Autodesk Fusion 360 part; units mm, degrees
(part 3 of 4)
sketch "SupportPlate" plane through (0, 0, 0) normal (0, 0, 1) x (1, 0, 0)
  line L0 (113.5494, -107.4434) -> (117.1134, -109.2589)
  spline S0 degree 3 poles (117.1134, -109.2589) (117.3594, -109.3843) (117.6605, -109.2865) (117.7859, -109.0398) knots 0 0 0 0 1 1 1 1
  line L1 (117.7859, -109.0398) -> (118.013, -108.5947)
  line L2 (118.013, -108.5947) -> (121.5769, -110.4103)
  spline S1 degree 3 poles (121.5769, -110.4103) (121.8229, -110.5362) (122.124, -110.4384) (122.2494, -110.1926) knots 0 0 0 0 1 1 1 1
  line L3 (122.2494, -110.1926) -> (128.1513, -98.6093)
  spline S2 degree 3 poles (128.1513, -98.6093) (128.2766, -98.3632) (128.1788, -98.0621) (127.9328, -97.937) knots 0 0 0 0 1 1 1 1
  line L4 (127.9328, -97.937) -> (124.3688, -96.1196)
  line L5 (124.3688, -96.1196) -> (124.5958, -95.6752)
  spline S3 degree 3 poles (124.5958, -95.6752) (124.7211, -95.4293) (124.6233, -95.1282) (124.3773, -95.0029) knots 0 0 0 0 1 1 1 1
  line L6 (124.3773, -95.0029) -> (120.8133, -93.1874)
  spline S4 degree 3 poles (120.8133, -93.1874) (120.5672, -93.0615) (120.2661, -93.1593) (120.1407, -93.4052) knots 0 0 0 0 1 1 1 1
  line L7 (120.1407, -93.4052) -> (119.9137, -93.8521)
  line L8 (119.9137, -93.8521) -> (116.3497, -92.0347)
  spline S5 degree 3 poles (116.3497, -92.0347) (116.1036, -91.9095) (115.8026, -92.0074) (115.6772, -92.2537) knots 0 0 0 0 1 1 1 1
  line L9 (115.6772, -92.2537) -> (109.7754, -103.837)
  spline S6 degree 3 poles (109.7754, -103.837) (109.6499, -104.0825) (109.7478, -104.3836) (109.9938, -104.5093) knots 0 0 0 0 1 1 1 1
  line L10 (109.9938, -104.5093) -> (113.5579, -106.3246)
  line L11 (113.5579, -106.3246) -> (113.3309, -106.7711)
  spline S7 degree 3 poles (113.3309, -106.7711) (113.2055, -107.0165) (113.3033, -107.3176) (113.5494, -107.4434) knots 0 0 0 0 1 1 1 1
  line L12 (129.9703, -110.4119) -> (133.5342, -112.2274)
  line L13 (133.5342, -112.2274) -> (133.3072, -112.6724)
  spline S8 degree 3 poles (133.3072, -112.6724) (133.1819, -112.9189) (133.2797, -113.22) (133.5258, -113.346) knots 0 0 0 0 1 1 1 1
  line L14 (133.5258, -113.346) -> (137.0897, -115.1615)
  spline S9 degree 3 poles (137.0897, -115.1615) (137.3358, -115.2867) (137.6369, -115.1889) (137.7623, -114.9424) knots 0 0 0 0 1 1 1 1
  line L15 (137.7623, -114.9424) -> (137.9893, -114.4975)
  line L16 (137.9893, -114.4975) -> (141.5533, -116.3129)
  spline S10 degree 3 poles (141.5533, -116.3129) (141.7994, -116.4387) (142.1004, -116.3408) (142.2258, -116.0952) knots 0 0 0 0 1 1 1 1
  line L17 (142.2258, -116.0952) -> (148.1276, -104.5119)
  spline S11 degree 3 poles (148.1276, -104.5119) (148.253, -104.2656) (148.1552, -103.9646) (147.9091, -103.8397) knots 0 0 0 0 1 1 1 1
  line L18 (147.9091, -103.8397) -> (144.3451, -102.0224)
  line L19 (144.3451, -102.0224) -> (144.5721, -101.5778)
  spline S12 degree 3 poles (144.5721, -101.5778) (144.6975, -101.3317) (144.5997, -101.0306) (144.3536, -100.9056) knots 0 0 0 0 1 1 1 1
  line L20 (144.3536, -100.9056) -> (140.7896, -99.0887)
  spline S13 degree 3 poles (140.7896, -99.0887) (140.5436, -98.9639) (140.2425, -99.0617) (140.1171, -99.3078) knots 0 0 0 0 1 1 1 1
  line L21 (140.1171, -99.3078) -> (139.8901, -99.7523)
  line L22 (139.8901, -99.7523) -> (136.3261, -97.9373)
  spline S14 degree 3 poles (136.3261, -97.9373) (136.08, -97.812) (135.779, -97.9098) (135.6536, -98.1564) knots 0 0 0 0 1 1 1 1
  line L23 (135.6536, -98.1564) -> (129.7517, -109.7383)
  spline S15 degree 3 poles (129.7517, -109.7383) (129.6264, -109.985) (129.7242, -110.2861) (129.9703, -110.4119) knots 0 0 0 0 1 1 1 1
  line L24 (99.4151, -97.8124) -> (99.4152, -97.3129)
  line L25 (99.4152, -97.3129) -> (103.4151, -97.3123)
  spline S16 degree 3 poles (103.4151, -97.3123) (103.6912, -97.3118) (103.9151, -97.088) (103.9151, -96.8123) knots 0 0 0 0 1 1 1 1
  line L26 (103.9151, -96.8123) -> (103.9151, -83.8115)
  spline S17 degree 3 poles (103.9151, -83.8115) (103.9151, -83.5357) (103.6912, -83.3118) (103.4151, -83.3114) knots 0 0 0 0 1 1 1 1
  line L27 (103.4151, -83.3114) -> (99.4152, -83.3112)
  line L28 (99.4152, -83.3112) -> (99.4151, -82.8115)
  spline S18 degree 3 poles (99.4151, -82.8115) (99.4151, -82.5358) (99.1912, -82.312) (98.9151, -82.3115) knots 0 0 0 0 1 1 1 1
  line L29 (98.9151, -82.3115) -> (94.9151, -82.3115)
  spline S19 degree 3 poles (94.9151, -82.3115) (94.639, -82.312) (94.4151, -82.5358) (94.4151, -82.8115) knots 0 0 0 0 1 1 1 1
  line L30 (94.4151, -82.8115) -> (94.4151, -83.3112)
  line L31 (94.4151, -83.3112) -> (90.4151, -83.3114)
  spline S20 degree 3 poles (90.4151, -83.3114) (90.139, -83.3117) (89.9151, -83.5357) (89.9151, -83.8115) knots 0 0 0 0 1 1 1 1
  line L32 (89.9151, -83.8115) -> (89.9151, -96.8123)
  spline S21 degree 3 poles (89.9151, -96.8123) (89.9151, -97.088) (90.139, -97.3119) (90.4151, -97.3123) knots 0 0 0 0 1 1 1 1
  line L33 (90.4151, -97.3123) -> (94.4151, -97.3129)
  line L34 (94.4151, -97.3129) -> (94.4151, -97.8124)
  spline S22 degree 3 poles (94.4151, -97.8124) (94.4151, -98.088) (94.639, -98.3119) (94.9151, -98.3124) knots 0 0 0 0 1 1 1 1
  line L35 (94.9151, -98.3124) -> (98.9151, -98.3124)
  spline S23 degree 3 poles (98.9151, -98.3124) (99.1912, -98.3119) (99.4151, -98.088) (99.4151, -97.8124) knots 0 0 0 0 1 1 1 1
  line L36 (61.3151, -97.8124) -> (61.3152, -97.3129)
  line L37 (61.3152, -97.3129) -> (65.3151, -97.3123)
  spline S24 degree 3 poles (65.3151, -97.3123) (65.5912, -97.3118) (65.8151, -97.088) (65.8152, -96.8123) knots 0 0 0 0 1 1 1 1
  line L38 (65.8152, -96.8123) -> (65.8152, -83.8115)
  spline S25 degree 3 poles (65.8152, -83.8115) (65.8151, -83.5357) (65.5912, -83.3118) (65.3151, -83.3114) knots 0 0 0 0 1 1 1 1
  line L39 (65.3151, -83.3114) -> (61.3152, -83.3112)
  line L40 (61.3152, -83.3112) -> (61.3151, -82.8115)
  spline S26 degree 3 poles (61.3151, -82.8115) (61.3151, -82.5358) (61.0912, -82.312) (60.8151, -82.3115) knots 0 0 0 0 1 1 1 1
  line L41 (60.8151, -82.3115) -> (56.8151, -82.3115)
  spline S27 degree 3 poles (56.8151, -82.3115) (56.539, -82.312) (56.3151, -82.5358) (56.3151, -82.8115) knots 0 0 0 0 1 1 1 1
  line L42 (56.3151, -82.8115) -> (56.3151, -83.3112)
  line L43 (56.3151, -83.3112) -> (52.3151, -83.3114)
  spline S28 degree 3 poles (52.3151, -83.3114) (52.039, -83.3117) (51.8151, -83.5357) (51.8151, -83.8115) knots 0 0 0 0 1 1 1 1
  line L44 (51.8151, -83.8115) -> (51.8151, -96.8123)
  spline S29 degree 3 poles (51.8151, -96.8123) (51.8151, -97.088) (52.039, -97.3119) (52.3151, -97.3123) knots 0 0 0 0 1 1 1 1
  line L45 (52.3151, -97.3123) -> (56.3151, -97.3129)
  line L46 (56.3151, -97.3129) -> (56.3151, -97.8124)
  spline S30 degree 3 poles (56.3151, -97.8124) (56.3151, -98.088) (56.539, -98.3119) (56.8151, -98.3124) knots 0 0 0 0 1 1 1 1
  line L47 (56.8151, -98.3124) -> (60.8151, -98.3124)
  spline S31 degree 3 poles (60.8151, -98.3124) (61.0912, -98.3119) (61.3151, -98.088) (61.3151, -97.8124) knots 0 0 0 0 1 1 1 1
  line L48 (80.3651, -95.4312) -> (80.3652, -94.9316)
  line L49 (80.3652, -94.9316) -> (84.3651, -94.9311)
  spline S32 degree 3 poles (84.3651, -94.9311) (84.6412, -94.9305) (84.8651, -94.7067) (84.8652, -94.431) knots 0 0 0 0 1 1 1 1
  line L50 (84.8652, -94.431) -> (84.8652, -81.4302)
  spline S33 degree 3 poles (84.8652, -81.4302) (84.8651, -81.1545) (84.6413, -80.9306) (84.3651, -80.9302) knots 0 0 0 0 1 1 1 1
  line L51 (84.3651, -80.9302) -> (80.3652, -80.9299)
  line L52 (80.3652, -80.9299) -> (80.3651, -80.4303)
  spline S34 degree 3 poles (80.3651, -80.4303) (80.3651, -80.1546) (80.1412, -79.9307) (79.8651, -79.9303) knots 0 0 0 0 1 1 1 1
  line L53 (79.8651, -79.9303) -> (75.8651, -79.9303)
  spline S35 degree 3 poles (75.8651, -79.9303) (75.589, -79.9308) (75.3651, -80.1546) (75.3651, -80.4303) knots 0 0 0 0 1 1 1 1
  line L54 (75.3651, -80.4303) -> (75.3651, -80.9299)
  line L55 (75.3651, -80.9299) -> (71.3651, -80.9302)
  spline S36 degree 3 poles (71.3651, -80.9302) (71.089, -80.9305) (70.8651, -81.1545) (70.8651, -81.4302) knots 0 0 0 0 1 1 1 1
  line L56 (70.8651, -81.4302) -> (70.8651, -94.431)
  spline S37 degree 3 poles (70.8651, -94.431) (70.8651, -94.7067) (71.089, -94.9306) (71.3651, -94.9311) knots 0 0 0 0 1 1 1 1
  line L57 (71.3651, -94.9311) -> (75.3651, -94.9316)
  line L58 (75.3651, -94.9316) -> (75.3651, -95.4312)
  spline S38 degree 3 poles (75.3651, -95.4312) (75.3651, -95.7068) (75.589, -95.9306) (75.8651, -95.9312) knots 0 0 0 0 1 1 1 1
  line L59 (75.8651, -95.9312) -> (79.8651, -95.9312)
  spline S39 degree 3 poles (79.8651, -95.9312) (80.1412, -95.9307) (80.3651, -95.7068) (80.3651, -95.4312) knots 0 0 0 0 1 1 1 1
  line L60 (42.2651, -83.5249) -> (42.2652, -83.0254)
  line L61 (42.2652, -83.0254) -> (46.2651, -83.0248)
  spline S40 degree 3 poles (46.2651, -83.0248) (46.5412, -83.0243) (46.7651, -82.8005) (46.7651, -82.5248) knots 0 0 0 0 1 1 1 1
  line L62 (46.7651, -82.5248) -> (46.7651, -69.524)
  spline S41 degree 3 poles (46.7651, -69.524) (46.7651, -69.2482) (46.5412, -69.0243) (46.2651, -69.0239) knots 0 0 0 0 1 1 1 1
  line L63 (46.2651, -69.0239) -> (42.2652, -69.0237)
  line L64 (42.2652, -69.0237) -> (42.2651, -68.524)
  spline S42 degree 3 poles (42.2651, -68.524) (42.2651, -68.2483) (42.0412, -68.0245) (41.7651, -68.024) knots 0 0 0 0 1 1 1 1
  line L65 (41.7651, -68.024) -> (37.7651, -68.024)
  spline S43 degree 3 poles (37.7651, -68.024) (37.489, -68.0245) (37.2651, -68.2483) (37.2651, -68.524) knots 0 0 0 0 1 1 1 1
  line L66 (37.2651, -68.524) -> (37.2651, -69.0237)
  line L67 (37.2651, -69.0237) -> (33.2651, -69.0239)
  spline S44 degree 3 poles (33.2651, -69.0239) (32.989, -69.0242) (32.7651, -69.2482) (32.7651, -69.524) knots 0 0 0 0 1 1 1 1
  line L68 (32.7651, -69.524) -> (32.7651, -82.5248)
  spline S45 degree 3 poles (32.7651, -82.5248) (32.7651, -82.8005) (32.989, -83.0244) (33.2651, -83.0248) knots 0 0 0 0 1 1 1 1
  line L69 (33.2651, -83.0248) -> (37.2651, -83.0254)
  line L70 (37.2651, -83.0254) -> (37.2651, -83.5249)
  spline S46 degree 3 poles (37.2651, -83.5249) (37.2651, -83.8005) (37.489, -84.0244) (37.7651, -84.0249) knots 0 0 0 0 1 1 1 1
  line L71 (37.7651, -84.0249) -> (41.7651, -84.0249)
  spline S47 degree 3 poles (41.7651, -84.0249) (42.0412, -84.0244) (42.2651, -83.8005) (42.2651, -83.5249) knots 0 0 0 0 1 1 1 1
  spline S48 degree 3 poles (17.9526, -84.0249) (18.2287, -84.0244) (18.4526, -83.8005) (18.4526, -83.5249) knots 0 0 0 0 1 1 1 1
  line L72 (18.4526, -83.5249) -> (18.4526, -83.0254)
  line L73 (18.4526, -83.0254) -> (22.4526, -83.0248)
  spline S49 degree 3 poles (22.4526, -83.0248) (22.7287, -83.0243) (22.9526, -82.8005) (22.9526, -82.5248) knots 0 0 0 0 1 1 1 1
  line L74 (22.9526, -82.5248) -> (22.9526, -69.524)
  spline S50 degree 3 poles (22.9526, -69.524) (22.9526, -69.2482) (22.7287, -69.0243) (22.4526, -69.0239) knots 0 0 0 0 1 1 1 1
  line L75 (22.4526, -69.0239) -> (18.4526, -69.0236)
  line L76 (18.4526, -69.0236) -> (18.4526, -68.524)
  spline S51 degree 3 poles (18.4526, -68.524) (18.4526, -68.2483) (18.2287, -68.0244) (17.9526, -68.0239) knots 0 0 0 0 1 1 1 1
  line L77 (17.9526, -68.0239) -> (13.9526, -68.0239)
  spline S52 degree 3 poles (13.9526, -68.0239) (13.6765, -68.0245) (13.4526, -68.2483) (13.4526, -68.524) knots 0 0 0 0 1 1 1 1
  line L78 (13.4526, -68.524) -> (13.4526, -69.0236)
  line L79 (13.4526, -69.0236) -> (9.4526, -69.0239)
  spline S53 degree 3 poles (9.4526, -69.0239) (9.1765, -69.0241) (8.9526, -69.2481) (8.9526, -69.5239) knots 0 0 0 0 1 1 1 1
  line L80 (8.9526, -69.5239) -> (8.9526, -82.5247)
  spline S54 degree 3 poles (8.9526, -82.5247) (8.9526, -82.8004) (9.1765, -83.0243) (9.4526, -83.0247) knots 0 0 0 0 1 1 1 1
  line L81 (9.4526, -83.0247) -> (13.4526, -83.0253)
  line L82 (13.4526, -83.0253) -> (13.4526, -83.5248)
  spline S55 degree 3 poles (13.4526, -83.5248) (13.4526, -83.8005) (13.6765, -84.0243) (13.9526, -84.0249) knots 0 0 0 0 1 1 1 1
  line L83 (13.9526, -84.0249) -> (17.9526, -84.0249)
  line L84 (118.4651, -81.1437) -> (118.4652, -80.6441)
  line L85 (118.4652, -80.6441) -> (122.4651, -80.6436)
  spline S56 degree 3 poles (122.4651, -80.6436) (122.7412, -80.643) (122.9651, -80.4192) (122.9651, -80.1435) knots 0 0 0 0 1 1 1 1
  line L86 (122.9651, -80.1435) -> (122.9651, -67.1427)
  spline S57 degree 3 poles (122.9651, -67.1427) (122.9651, -66.867) (122.7412, -66.6431) (122.4651, -66.6427) knots 0 0 0 0 1 1 1 1
  line L87 (122.4651, -66.6427) -> (118.4652, -66.6422)
  line L88 (118.4652, -66.6422) -> (118.4651, -66.1425)
  spline S58 degree 3 poles (118.4651, -66.1425) (118.4651, -65.8668) (118.2412, -65.643) (117.9651, -65.6425) knots 0 0 0 0 1 1 1 1
  line L89 (117.9651, -65.6425) -> (113.9651, -65.6425)
  spline S59 degree 3 poles (113.9651, -65.6425) (113.689, -65.643) (113.4651, -65.8668) (113.4651, -66.1425) knots 0 0 0 0 1 1 1 1
  line L90 (113.4651, -66.1425) -> (113.4651, -66.6422)
  line L91 (113.4651, -66.6422) -> (109.4651, -66.6427)
  spline S60 degree 3 poles (109.4651, -66.6427) (109.189, -66.643) (108.9651, -66.867) (108.9651, -67.1427) knots 0 0 0 0 1 1 1 1
  line L92 (108.9651, -67.1427) -> (108.9651, -80.1435)
  spline S61 degree 3 poles (108.9651, -80.1435) (108.9651, -80.4192) (109.189, -80.6431) (109.4651, -80.6436) knots 0 0 0 0 1 1 1 1
  line L93 (109.4651, -80.6436) -> (113.4651, -80.6441)
  line L94 (113.4651, -80.6441) -> (113.4651, -81.1437)
  spline S62 degree 3 poles (113.4651, -81.1437) (113.4651, -81.4193) (113.689, -81.6431) (113.9651, -81.6437) knots 0 0 0 0 1 1 1 1
  line L95 (113.9651, -81.6437) -> (117.9651, -81.6437)
  spline S63 degree 3 poles (117.9651, -81.6437) (118.2412, -81.6432) (118.4651, -81.4193) (118.4651, -81.1437) knots 0 0 0 0 1 1 1 1
  line L96 (99.4151, -78.7624) -> (99.4152, -78.2629)
  line L97 (99.4152, -78.2629) -> (103.4151, -78.2623)
  spline S64 degree 3 poles (103.4151, -78.2623) (103.6912, -78.2618) (103.9151, -78.038) (103.9151, -77.7623) knots 0 0 0 0 1 1 1 1
  line L98 (103.9151, -77.7623) -> (103.9151, -64.7615)
  spline S65 degree 3 poles (103.9151, -64.7615) (103.9151, -64.4857) (103.6912, -64.2618) (103.4151, -64.2615) knots 0 0 0 0 1 1 1 1
  line L99 (103.4151, -64.2615) -> (99.4152, -64.2609)
  line L100 (99.4152, -64.2609) -> (99.4151, -63.7613)
  spline S66 degree 3 poles (99.4151, -63.7613) (99.4151, -63.4856) (99.1912, -63.2617) (98.9151, -63.2613) knots 0 0 0 0 1 1 1 1
  line L101 (98.9151, -63.2613) -> (94.9151, -63.2613)
  spline S67 degree 3 poles (94.9151, -63.2613) (94.639, -63.2618) (94.4151, -63.4856) (94.4151, -63.7613) knots 0 0 0 0 1 1 1 1
  line L102 (94.4151, -63.7613) -> (94.4151, -64.2609)
  line L103 (94.4151, -64.2609) -> (90.4151, -64.2615)
  spline S68 degree 3 poles (90.4151, -64.2615) (90.139, -64.2617) (89.9151, -64.4857) (89.9151, -64.7615) knots 0 0 0 0 1 1 1 1
  line L104 (89.9151, -64.7615) -> (89.9151, -77.7623)
  spline S69 degree 3 poles (89.9151, -77.7623) (89.9151, -78.038) (90.139, -78.2619) (90.4151, -78.2623) knots 0 0 0 0 1 1 1 1
  line L105 (90.4151, -78.2623) -> (94.4151, -78.2629)
  line L106 (94.4151, -78.2629) -> (94.4151, -78.7624)
  spline S70 degree 3 poles (94.4151, -78.7624) (94.4151, -79.038) (94.639, -79.2619) (94.9151, -79.2624) knots 0 0 0 0 1 1 1 1
  line L107 (94.9151, -79.2624) -> (98.9151, -79.2624)
  spline S71 degree 3 poles (98.9151, -79.2624) (99.1912, -79.2619) (99.4151, -79.038) (99.4151, -78.7624) knots 0 0 0 0 1 1 1 1
  line L108 (61.3151, -78.7624) -> (61.3152, -78.2629)
  line L109 (61.3152, -78.2629) -> (65.3151, -78.2623)
  spline S72 degree 3 poles (65.3151, -78.2623) (65.5912, -78.2618) (65.8151, -78.038) (65.8152, -77.7623) knots 0 0 0 0 1 1 1 1
  line L110 (65.8152, -77.7623) -> (65.8152, -64.7615)
  spline S73 degree 3 poles (65.8152, -64.7615) (65.8151, -64.4857) (65.5912, -64.2618) (65.3151, -64.2615) knots 0 0 0 0 1 1 1 1
  line L111 (65.3151, -64.2615) -> (61.3152, -64.2609)
  line L112 (61.3152, -64.2609) -> (61.3151, -63.7613)
  spline S74 degree 3 poles (61.3151, -63.7613) (61.3151, -63.4856) (61.0912, -63.2617) (60.8151, -63.2613) knots 0 0 0 0 1 1 1 1
  line L113 (60.8151, -63.2613) -> (56.8151, -63.2613)
  spline S75 degree 3 poles (56.8151, -63.2613) (56.539, -63.2618) (56.3151, -63.4856) (56.3151, -63.7613) knots 0 0 0 0 1 1 1 1
  line L114 (56.3151, -63.7613) -> (56.3151, -64.2609)
  line L115 (56.3151, -64.2609) -> (52.3151, -64.2615)
  spline S76 degree 3 poles (52.3151, -64.2615) (52.039, -64.2617) (51.8151, -64.4857) (51.8151, -64.7615) knots 0 0 0 0 1 1 1 1
  line L116 (51.8151, -64.7615) -> (51.8151, -77.7623)
  spline S77 degree 3 poles (51.8151, -77.7623) (51.8151, -78.038) (52.039, -78.2619) (52.3151, -78.2623) knots 0 0 0 0 1 1 1 1
  line L117 (52.3151, -78.2623) -> (56.3151, -78.2629)
  line L118 (56.3151, -78.2629) -> (56.3151, -78.7624)
  spline S78 degree 3 poles (56.3151, -78.7624) (56.3151, -79.038) (56.539, -79.2619) (56.8151, -79.2624) knots 0 0 0 0 1 1 1 1
  line L119 (56.8151, -79.2624) -> (60.8151, -79.2624)
  spline S79 degree 3 poles (60.8151, -79.2624) (61.0912, -79.2619) (61.3151, -79.038) (61.3151, -78.7624) knots 0 0 0 0 1 1 1 1
  line L120 (80.3651, -76.3812) -> (80.3652, -75.8816)
  line L121 (80.3652, -75.8816) -> (84.3651, -75.8811)
  spline S80 degree 3 poles (84.3651, -75.8811) (84.6412, -75.8805) (84.8651, -75.6567) (84.8652, -75.381) knots 0 0 0 0 1 1 1 1
  line L122 (84.8652, -75.381) -> (84.8652, -62.3802)
  spline S81 degree 3 poles (84.8652, -62.3802) (84.8651, -62.1045) (84.6413, -61.8806) (84.3651, -61.8802) knots 0 0 0 0 1 1 1 1
  line L123 (84.3651, -61.8802) -> (80.3652, -61.8797)
  line L124 (80.3652, -61.8797) -> (80.3651, -61.38)
  spline S82 degree 3 poles (80.3651, -61.38) (80.3651, -61.1043) (80.1412, -60.8805) (79.8651, -60.88) knots 0 0 0 0 1 1 1 1
  line L125 (79.8651, -60.88) -> (75.8651, -60.88)
  spline S83 degree 3 poles (75.8651, -60.88) (75.589, -60.8805) (75.3651, -61.1043) (75.3651, -61.38) knots 0 0 0 0 1 1 1 1
  line L126 (75.3651, -61.38) -> (75.3651, -61.8797)
  line L127 (75.3651, -61.8797) -> (71.3651, -61.8802)
  spline S84 degree 3 poles (71.3651, -61.8802) (71.089, -61.8805) (70.8651, -62.1045) (70.8651, -62.3802) knots 0 0 0 0 1 1 1 1
  line L128 (70.8651, -62.3802) -> (70.8651, -75.381)
  spline S85 degree 3 poles (70.8651, -75.381) (70.8651, -75.6567) (71.089, -75.8806) (71.3651, -75.8811) knots 0 0 0 0 1 1 1 1
  line L129 (71.3651, -75.8811) -> (75.3651, -75.8816)
  line L130 (75.3651, -75.8816) -> (75.3651, -76.3812)
  spline S86 degree 3 poles (75.3651, -76.3812) (75.3651, -76.6568) (75.589, -76.8806) (75.8651, -76.8812) knots 0 0 0 0 1 1 1 1
  line L131 (75.8651, -76.8812) -> (79.8651, -76.8812)
  spline S87 degree 3 poles (79.8651, -76.8812) (80.1412, -76.8807) (80.3651, -76.6568) (80.3651, -76.3812) knots 0 0 0 0 1 1 1 1
  line L132 (137.5151, -71.6187) -> (137.5152, -71.1191)
  line L133 (137.5152, -71.1191) -> (141.5151, -71.1186)
  spline S88 degree 3 poles (141.5151, -71.1186) (141.7912, -71.118) (142.0151, -70.8942) (142.0152, -70.6185) knots 0 0 0 0 1 1 1 1
  line L134 (142.0152, -70.6185) -> (142.0152, -57.6177)
  spline S89 degree 3 poles (142.0152, -57.6177) (142.0151, -57.342) (141.7912, -57.1181) (141.5151, -57.1177) knots 0 0 0 0 1 1 1 1
  line L135 (141.5151, -57.1177) -> (137.5152, -57.1172)
  line L136 (137.5152, -57.1172) -> (137.5151, -56.6175)
  spline S90 degree 3 poles (137.5151, -56.6175) (137.5151, -56.3418) (137.2913, -56.118) (137.0151, -56.1175) knots 0 0 0 0 1 1 1 1
  line L137 (137.0151, -56.1175) -> (133.0151, -56.1175)
  spline S91 degree 3 poles (133.0151, -56.1175) (132.739, -56.118) (132.5151, -56.3418) (132.5151, -56.6175) knots 0 0 0 0 1 1 1 1
  line L138 (132.5151, -56.6175) -> (132.5151, -57.1172)
  line L139 (132.5151, -57.1172) -> (128.5151, -57.1177)
  spline S92 degree 3 poles (128.5151, -57.1177) (128.239, -57.118) (128.0151, -57.342) (128.0151, -57.6177) knots 0 0 0 0 1 1 1 1
  line L140 (128.0151, -57.6177) -> (128.0151, -70.6185)
  spline S93 degree 3 poles (128.0151, -70.6185) (128.0151, -70.8942) (128.239, -71.1181) (128.5151, -71.1186) knots 0 0 0 0 1 1 1 1
  line L141 (128.5151, -71.1186) -> (132.5151, -71.1191)
  line L142 (132.5151, -71.1191) -> (132.5151, -71.6187)
  spline S94 degree 3 poles (132.5151, -71.6187) (132.5151, -71.8943) (132.739, -72.1181) (133.0151, -72.1187) knots 0 0 0 0 1 1 1 1
  line L143 (133.0151, -72.1187) -> (137.0151, -72.1187)
  spline S95 degree 3 poles (137.0151, -72.1187) (137.2912, -72.1182) (137.5151, -71.8943) (137.5151, -71.6187) knots 0 0 0 0 1 1 1 1
  line L144 (42.2651, -64.4749) -> (42.2652, -63.9754)
  line L145 (42.2652, -63.9754) -> (46.2651, -63.9748)
  spline S96 degree 3 poles (46.2651, -63.9748) (46.5413, -63.9743) (46.7651, -63.7505) (46.7652, -63.4748) knots 0 0 0 0 1 1 1 1
  line L146 (46.7652, -63.4748) -> (46.7652, -50.474)
  spline S97 degree 3 poles (46.7652, -50.474) (46.7651, -50.1982) (46.5413, -49.9743) (46.2651, -49.974) knots 0 0 0 0 1 1 1 1
  line L147 (46.2651, -49.974) -> (42.2652, -49.9734)
  line L148 (42.2652, -49.9734) -> (42.2651, -49.4738)
  spline S98 degree 3 poles (42.2651, -49.4738) (42.2651, -49.1981) (42.0413, -48.9742) (41.7651, -48.9738) knots 0 0 0 0 1 1 1 1
  line L149 (41.7651, -48.9738) -> (37.7651, -48.9738)
  spline S99 degree 3 poles (37.7651, -48.9738) (37.489, -48.9743) (37.2651, -49.1981) (37.2651, -49.4738) knots 0 0 0 0 1 1 1 1
  line L150 (37.2651, -49.4738) -> (37.2651, -49.9734)
  line L151 (37.2651, -49.9734) -> (33.2651, -49.974)
  spline S100 degree 3 poles (33.2651, -49.974) (32.989, -49.9742) (32.7651, -50.1982) (32.7651, -50.474) knots 0 0 0 0 1 1 1 1
  line L152 (32.7651, -50.474) -> (32.7651, -63.4748)
  spline S101 degree 3 poles (32.7651, -63.4748) (32.7651, -63.7505) (32.989, -63.9743) (33.2651, -63.9748) knots 0 0 0 0 1 1 1 1
  line L153 (33.2651, -63.9748) -> (37.2651, -63.9754)
  line L154 (37.2651, -63.9754) -> (37.2651, -64.4749)
  spline S102 degree 3 poles (37.2651, -64.4749) (37.2651, -64.7505) (37.489, -64.9744) (37.7651, -64.9749) knots 0 0 0 0 1 1 1 1
  line L155 (37.7651, -64.9749) -> (41.7651, -64.9749)
  spline S103 degree 3 poles (41.7651, -64.9749) (42.0413, -64.9744) (42.2651, -64.7505) (42.2651, -64.4749) knots 0 0 0 0 1 1 1 1
  spline S104 degree 3 poles (17.9526, -64.9749) (18.2288, -64.9744) (18.4526, -64.7505) (18.4526, -64.4749) knots 0 0 0 0 1 1 1 1
  line L156 (18.4526, -64.4749) -> (18.4526, -63.9754)
  line L157 (18.4526, -63.9754) -> (22.4526, -63.9748)
  spline S105 degree 3 poles (22.4526, -63.9748) (22.7288, -63.9743) (22.9526, -63.7505) (22.9526, -63.4748) knots 0 0 0 0 1 1 1 1
  line L158 (22.9526, -63.4748) -> (22.9526, -50.474)
  spline S106 degree 3 poles (22.9526, -50.474) (22.9526, -50.1982) (22.7288, -49.9743) (22.4526, -49.9739) knots 0 0 0 0 1 1 1 1
  line L159 (22.4526, -49.9739) -> (18.4526, -49.9736)
  line L160 (18.4526, -49.9736) -> (18.4526, -49.474)
  spline S107 degree 3 poles (18.4526, -49.474) (18.4526, -49.1983) (18.2287, -48.9744) (17.9526, -48.9739) knots 0 0 0 0 1 1 1 1
  line L161 (17.9526, -48.9739) -> (13.9526, -48.9739)
  spline S108 degree 3 poles (13.9526, -48.9739) (13.6765, -48.9745) (13.4526, -49.1983) (13.4526, -49.474) knots 0 0 0 0 1 1 1 1
  line L162 (13.4526, -49.474) -> (13.4526, -49.9736)
  line L163 (13.4526, -49.9736) -> (9.4526, -49.9739)
  spline S109 degree 3 poles (9.4526, -49.9739) (9.1765, -49.9741) (8.9526, -50.1981) (8.9526, -50.4739) knots 0 0 0 0 1 1 1 1
  line L164 (8.9526, -50.4739) -> (8.9526, -63.4747)
  spline S110 degree 3 poles (8.9526, -63.4747) (8.9526, -63.7504) (9.1765, -63.9743) (9.4526, -63.9747) knots 0 0 0 0 1 1 1 1
  line L165 (9.4526, -63.9747) -> (13.4526, -63.9753)
  line L166 (13.4526, -63.9753) -> (13.4526, -64.4748)
  spline S111 degree 3 poles (13.4526, -64.4748) (13.4526, -64.7505) (13.6765, -64.9743) (13.9526, -64.9749) knots 0 0 0 0 1 1 1 1
  line L167 (13.9526, -64.9749) -> (17.9526, -64.9749)
  line L168 (118.4651, -62.0937) -> (118.4652, -61.5941)
  line L169 (118.4652, -61.5941) -> (122.4651, -61.5936)
  spline S112 degree 3 poles (122.4651, -61.5936) (122.7413, -61.593) (122.9651, -61.3692) (122.9652, -61.0935) knots 0 0 0 0 1 1 1 1
  line L170 (122.9652, -61.0935) -> (122.9652, -48.0927)
  spline S113 degree 3 poles (122.9652, -48.0927) (122.9651, -47.817) (122.7413, -47.5931) (122.4651, -47.5927) knots 0 0 0 0 1 1 1 1
  line L171 (122.4651, -47.5927) -> (118.4652, -47.5922)
  line L172 (118.4652, -47.5922) -> (118.4651, -47.0925)
  spline S114 degree 3 poles (118.4651, -47.0925) (118.4651, -46.8168) (118.2413, -46.593) (117.9651, -46.5925) knots 0 0 0 0 1 1 1 1
  line L173 (117.9651, -46.5925) -> (113.9651, -46.5925)
  spline S115 degree 3 poles (113.9651, -46.5925) (113.689, -46.593) (113.4651, -46.8168) (113.4651, -47.0925) knots 0 0 0 0 1 1 1 1
  line L174 (113.4651, -47.0925) -> (113.4651, -47.5922)
  line L175 (113.4651, -47.5922) -> (109.4651, -47.5927)
  spline S116 degree 3 poles (109.4651, -47.5927) (109.189, -47.593) (108.9651, -47.817) (108.9651, -48.0927) knots 0 0 0 0 1 1 1 1
  line L176 (108.9651, -48.0927) -> (108.9651, -61.0935)
  spline S117 degree 3 poles (108.9651, -61.0935) (108.9651, -61.3692) (109.189, -61.5931) (109.4651, -61.5936) knots 0 0 0 0 1 1 1 1
  line L177 (109.4651, -61.5936) -> (113.4651, -61.5941)
  line L178 (113.4651, -61.5941) -> (113.4651, -62.0937)
  spline S118 degree 3 poles (113.4651, -62.0937) (113.4651, -62.3693) (113.689, -62.5931) (113.9651, -62.5937) knots 0 0 0 0 1 1 1 1
  line L179 (113.9651, -62.5937) -> (117.9651, -62.5937)
  spline S119 degree 3 poles (117.9651, -62.5937) (118.2412, -62.5932) (118.4651, -62.3693) (118.4651, -62.0937) knots 0 0 0 0 1 1 1 1
  line L180 (99.4151, -59.7124) -> (99.4152, -59.2129)
  line L181 (99.4152, -59.2129) -> (103.4151, -59.2123)
  spline S120 degree 3 poles (103.4151, -59.2123) (103.6913, -59.2118) (103.9151, -58.988) (103.9152, -58.7123) knots 0 0 0 0 1 1 1 1
  line L182 (103.9152, -58.7123) -> (103.9152, -45.7115)
  spline S121 degree 3 poles (103.9152, -45.7115) (103.9151, -45.4357) (103.6913, -45.2118) (103.4151, -45.2115) knots 0 0 0 0 1 1 1 1
  line L183 (103.4151, -45.2115) -> (99.4152, -45.2109)
  line L184 (99.4152, -45.2109) -> (99.4151, -44.7113)
  spline S122 degree 3 poles (99.4151, -44.7113) (99.4151, -44.4356) (99.1913, -44.2117) (98.9151, -44.2113) knots 0 0 0 0 1 1 1 1
  line L185 (98.9151, -44.2113) -> (94.9151, -44.2113)
  spline S123 degree 3 poles (94.9151, -44.2113) (94.639, -44.2118) (94.4151, -44.4356) (94.4151, -44.7113) knots 0 0 0 0 1 1 1 1
  line L186 (94.4151, -44.7113) -> (94.4151, -45.2109)
  line L187 (94.4151, -45.2109) -> (90.4151, -45.2115)
  spline S124 degree 3 poles (90.4151, -45.2115) (90.139, -45.2117) (89.9151, -45.4357) (89.9151, -45.7115) knots 0 0 0 0 1 1 1 1
  line L188 (89.9151, -45.7115) -> (89.9151, -58.7123)
  spline S125 degree 3 poles (89.9151, -58.7123) (89.9151, -58.988) (90.139, -59.2118) (90.4151, -59.2123) knots 0 0 0 0 1 1 1 1
  line L189 (90.4151, -59.2123) -> (94.4151, -59.2129)
  line L190 (94.4151, -59.2129) -> (94.4151, -59.7124)
  spline S126 degree 3 poles (94.4151, -59.7124) (94.4151, -59.988) (94.639, -60.2119) (94.9151, -60.2124) knots 0 0 0 0 1 1 1 1
  line L191 (94.9151, -60.2124) -> (98.9151, -60.2124)
  spline S127 degree 3 poles (98.9151, -60.2124) (99.1912, -60.2119) (99.4151, -59.988) (99.4151, -59.7124) knots 0 0 0 0 1 1 1 1
  line L192 (61.3151, -59.7124) -> (61.3152, -59.2129)
  line L193 (61.3152, -59.2129) -> (65.3151, -59.2123)
  spline S128 degree 3 poles (65.3151, -59.2123) (65.5913, -59.2118) (65.8151, -58.988) (65.8152, -58.7123) knots 0 0 0 0 1 1 1 1
  line L194 (65.8152, -58.7123) -> (65.8152, -45.7115)
  spline S129 degree 3 poles (65.8152, -45.7115) (65.8151, -45.4357) (65.5913, -45.2118) (65.3151, -45.2115) knots 0 0 0 0 1 1 1 1
  line L195 (65.3151, -45.2115) -> (61.3152, -45.2109)
  line L196 (61.3152, -45.2109) -> (61.3151, -44.7113)
  spline S130 degree 3 poles (61.3151, -44.7113) (61.3151, -44.4356) (61.0913, -44.2117) (60.8151, -44.2113) knots 0 0 0 0 1 1 1 1
  line L197 (60.8151, -44.2113) -> (56.8151, -44.2113)
  spline S131 degree 3 poles (56.8151, -44.2113) (56.539, -44.2118) (56.3151, -44.4356) (56.3151, -44.7113) knots 0 0 0 0 1 1 1 1
  line L198 (56.3151, -44.7113) -> (56.3151, -45.2109)
  line L199 (56.3151, -45.2109) -> (52.3151, -45.2115)
  spline S132 degree 3 poles (52.3151, -45.2115) (52.039, -45.2117) (51.8151, -45.4357) (51.8151, -45.7115) knots 0 0 0 0 1 1 1 1
  line L200 (51.8151, -45.7115) -> (51.8151, -58.7123)
  spline S133 degree 3 poles (51.8151, -58.7123) (51.8151, -58.988) (52.039, -59.2118) (52.3151, -59.2123) knots 0 0 0 0 1 1 1 1
  line L201 (52.3151, -59.2123) -> (56.3151, -59.2129)
  line L202 (56.3151, -59.2129) -> (56.3151, -59.7124)
  spline S134 degree 3 poles (56.3151, -59.7124) (56.3151, -59.988) (56.539, -60.2119) (56.8151, -60.2124) knots 0 0 0 0 1 1 1 1
  line L203 (56.8151, -60.2124) -> (60.8151, -60.2124)
  spline S135 degree 3 poles (60.8151, -60.2124) (61.0913, -60.2119) (61.3151, -59.988) (61.3151, -59.7124) knots 0 0 0 0 1 1 1 1
  line L204 (80.3651, -57.3312) -> (80.3652, -56.8316)
  line L205 (80.3652, -56.8316) -> (84.3651, -56.8311)
  spline S136 degree 3 poles (84.3651, -56.8311) (84.6413, -56.8305) (84.8651, -56.6067) (84.8652, -56.331) knots 0 0 0 0 1 1 1 1
  line L206 (84.8652, -56.331) -> (84.8652, -43.3302)
  spline S137 degree 3 poles (84.8652, -43.3302) (84.8651, -43.0545) (84.6413, -42.8306) (84.3651, -42.8302) knots 0 0 0 0 1 1 1 1
  line L207 (84.3651, -42.8302) -> (80.3652, -42.8297)
  line L208 (80.3652, -42.8297) -> (80.3651, -42.33)
  spline S138 degree 3 poles (80.3651, -42.33) (80.3651, -42.0543) (80.1413, -41.8305) (79.8651, -41.83) knots 0 0 0 0 1 1 1 1
  line L209 (79.8651, -41.83) -> (75.8651, -41.83)
  spline S139 degree 3 poles (75.8651, -41.83) (75.589, -41.8305) (75.3651, -42.0543) (75.3651, -42.33) knots 0 0 0 0 1 1 1 1
  line L210 (75.3651, -42.33) -> (75.3651, -42.8297)
  line L211 (75.3651, -42.8297) -> (71.3651, -42.8302)
  spline S140 degree 3 poles (71.3651, -42.8302) (71.089, -42.8305) (70.8651, -43.0545) (70.8651, -43.3302) knots 0 0 0 0 1 1 1 1
  line L212 (70.8651, -43.3302) -> (70.8651, -56.331)
  spline S141 degree 3 poles (70.8651, -56.331) (70.8651, -56.6067) (71.089, -56.8306) (71.3651, -56.8311) knots 0 0 0 0 1 1 1 1
  line L213 (71.3651, -56.8311) -> (75.3651, -56.8316)
  line L214 (75.3651, -56.8316) -> (75.3651, -57.3312)
  spline S142 degree 3 poles (75.3651, -57.3312) (75.3651, -57.6068) (75.589, -57.8306) (75.8651, -57.8312) knots 0 0 0 0 1 1 1 1
  line L215 (75.8651, -57.8312) -> (79.8651, -57.8312)
  spline S143 degree 3 poles (79.8651, -57.8312) (80.1412, -57.8307) (80.3651, -57.6068) (80.3651, -57.3312) knots 0 0 0 0 1 1 1 1
  line L216 (42.2651, -45.4249) -> (42.2652, -44.9254)
  line L217 (42.2652, -44.9254) -> (46.2651, -44.9248)
  spline S144 degree 3 poles (46.2651, -44.9248) (46.5413, -44.9243) (46.7651, -44.7005) (46.7652, -44.4248) knots 0 0 0 0 1 1 1 1
  line L218 (46.7652, -44.4248) -> (46.7652, -31.424)
  spline S145 degree 3 poles (46.7652, -31.424) (46.7651, -31.1482) (46.5413, -30.9243) (46.2651, -30.9239) knots 0 0 0 0 1 1 1 1
  line L219 (46.2651, -30.9239) -> (42.2652, -30.9237)
  line L220 (42.2652, -30.9237) -> (42.2651, -30.4241)
  spline S146 degree 3 poles (42.2651, -30.4241) (42.2651, -30.1483) (42.0413, -29.9245) (41.7651, -29.924) knots 0 0 0 0 1 1 1 1
  line L221 (41.7651, -29.924) -> (37.7651, -29.924)
  spline S147 degree 3 poles (37.7651, -29.924) (37.489, -29.9245) (37.2651, -30.1483) (37.2651, -30.4241) knots 0 0 0 0 1 1 1 1
  line L222 (37.2651, -30.4241) -> (37.2651, -30.9237)
  line L223 (37.2651, -30.9237) -> (33.2651, -30.9239)
  spline S148 degree 3 poles (33.2651, -30.9239) (32.989, -30.9245) (32.7651, -31.1482) (32.7651, -31.424) knots 0 0 0 0 1 1 1 1
  line L224 (32.7651, -31.424) -> (32.7651, -44.4248)
  spline S149 degree 3 poles (32.7651, -44.4248) (32.7651, -44.7005) (32.989, -44.9243) (33.2651, -44.9248) knots 0 0 0 0 1 1 1 1
  line L225 (33.2651, -44.9248) -> (37.2651, -44.9254)
  line L226 (37.2651, -44.9254) -> (37.2651, -45.4249)
  spline S150 degree 3 poles (37.2651, -45.4249) (37.2651, -45.7005) (37.489, -45.9244) (37.7651, -45.9249) knots 0 0 0 0 1 1 1 1
  line L227 (37.7651, -45.9249) -> (41.7651, -45.9249)
  spline S151 degree 3 poles (41.7651, -45.9249) (42.0413, -45.9244) (42.2651, -45.7005) (42.2651, -45.4249) knots 0 0 0 0 1 1 1 1
  spline S152 degree 3 poles (17.9526, -45.9249) (18.2288, -45.9244) (18.4526, -45.7005) (18.4526, -45.4249) knots 0 0 0 0 1 1 1 1
  line L228 (18.4526, -45.4249) -> (18.4526, -44.9254)
  line L229 (18.4526, -44.9254) -> (22.4526, -44.9248)
  spline S153 degree 3 poles (22.4526, -44.9248) (22.7288, -44.9243) (22.9526, -44.7005) (22.9526, -44.4248) knots 0 0 0 0 1 1 1 1
  line L230 (22.9526, -44.4248) -> (22.9526, -31.424)
  spline S154 degree 3 poles (22.9526, -31.424) (22.9526, -31.1482) (22.7288, -30.9243) (22.4526, -30.9239) knots 0 0 0 0 1 1 1 1
  line L231 (22.4526, -30.9239) -> (18.4526, -30.9236)
  line L232 (18.4526, -30.9236) -> (18.4526, -30.424)
  spline S155 degree 3 poles (18.4526, -30.424) (18.4526, -30.1483) (18.2287, -29.9244) (17.9526, -29.9239) knots 0 0 0 0 1 1 1 1
  line L233 (17.9526, -29.9239) -> (13.9526, -29.9239)
  spline S156 degree 3 poles (13.9526, -29.9239) (13.6765, -29.9245) (13.4526, -30.1483) (13.4526, -30.424) knots 0 0 0 0 1 1 1 1
  line L234 (13.4526, -30.424) -> (13.4526, -30.9236)
  line L235 (13.4526, -30.9236) -> (9.4526, -30.9239)
  spline S157 degree 3 poles (9.4526, -30.9239) (9.1765, -30.9244) (8.9526, -31.1481) (8.9526, -31.4239) knots 0 0 0 0 1 1 1 1
  line L236 (8.9526, -31.4239) -> (8.9526, -44.4247)
  spline S158 degree 3 poles (8.9526, -44.4247) (8.9526, -44.7004) (9.1765, -44.9243) (9.4526, -44.9247) knots 0 0 0 0 1 1 1 1
  line L237 (9.4526, -44.9247) -> (13.4526, -44.9253)
  line L238 (13.4526, -44.9253) -> (13.4526, -45.4248)
  spline S159 degree 3 poles (13.4526, -45.4248) (13.4526, -45.7005) (13.6765, -45.9243) (13.9526, -45.9249) knots 0 0 0 0 1 1 1 1
  line L239 (13.9526, -45.9249) -> (17.9526, -45.9249)
  line L240 (118.4651, -43.0437) -> (118.4652, -42.5441)
  line L241 (118.4652, -42.5441) -> (122.4651, -42.5436)
  spline S160 degree 3 poles (122.4651, -42.5436) (122.7413, -42.543) (122.9651, -42.3192) (122.9652, -42.0435) knots 0 0 0 0 1 1 1 1
  line L242 (122.9652, -42.0435) -> (122.9652, -29.0427)
  spline S161 degree 3 poles (122.9652, -29.0427) (122.9651, -28.767) (122.7413, -28.5431) (122.4651, -28.5427) knots 0 0 0 0 1 1 1 1
  line L243 (122.4651, -28.5427) -> (118.4652, -28.5424)
  line L244 (118.4652, -28.5424) -> (118.4651, -28.0428)
  spline S162 degree 3 poles (118.4651, -28.0428) (118.4651, -27.7671) (118.2413, -27.5432) (117.9651, -27.5428) knots 0 0 0 0 1 1 1 1
  line L245 (117.9651, -27.5428) -> (113.9651, -27.5428)
  spline S163 degree 3 poles (113.9651, -27.5428) (113.689, -27.5432) (113.4651, -27.7671) (113.4651, -28.0428) knots 0 0 0 0 1 1 1 1
  line L246 (113.4651, -28.0428) -> (113.4651, -28.5424)
  line L247 (113.4651, -28.5424) -> (109.4651, -28.5427)
  spline S164 degree 3 poles (109.4651, -28.5427) (109.189, -28.5432) (108.9651, -28.767) (108.9651, -29.0427) knots 0 0 0 0 1 1 1 1
  line L248 (108.9651, -29.0427) -> (108.9651, -42.0435)
  spline S165 degree 3 poles (108.9651, -42.0435) (108.9651, -42.3192) (109.189, -42.5431) (109.4651, -42.5436) knots 0 0 0 0 1 1 1 1
  line L249 (109.4651, -42.5436) -> (113.4651, -42.5441)
  line L250 (113.4651, -42.5441) -> (113.4651, -43.0437)
  spline S166 degree 3 poles (113.4651, -43.0437) (113.4651, -43.3193) (113.689, -43.5431) (113.9651, -43.5437) knots 0 0 0 0 1 1 1 1
  line L251 (113.9651, -43.5437) -> (117.9651, -43.5437)
  spline S167 degree 3 poles (117.9651, -43.5437) (118.2412, -43.5432) (118.4651, -43.3193) (118.4651, -43.0437) knots 0 0 0 0 1 1 1 1
  line L252 (99.4151, -40.6624) -> (99.4152, -40.1629)
  line L253 (99.4152, -40.1629) -> (103.4151, -40.1623)
  spline S168 degree 3 poles (103.4151, -40.1623) (103.6913, -40.1618) (103.9151, -39.938) (103.9152, -39.6623) knots 0 0 0 0 1 1 1 1
  line L254 (103.9152, -39.6623) -> (103.9152, -26.6615)
  spline S169 degree 3 poles (103.9152, -26.6615) (103.9151, -26.3858) (103.6913, -26.1619) (103.4151, -26.1615) knots 0 0 0 0 1 1 1 1
  line L255 (103.4151, -26.1615) -> (99.4152, -26.1611)
  line L256 (99.4152, -26.1611) -> (99.4151, -25.6615)
  spline S170 degree 3 poles (99.4151, -25.6615) (99.4151, -25.3858) (99.1912, -25.1619) (98.9151, -25.1614) knots 0 0 0 0 1 1 1 1
  line L257 (98.9151, -25.1614) -> (94.9151, -25.1614)
  spline S171 degree 3 poles (94.9151, -25.1614) (94.639, -25.1619) (94.4151, -25.3858) (94.4151, -25.6615) knots 0 0 0 0 1 1 1 1
  line L258 (94.4151, -25.6615) -> (94.415, -26.1611)
  line L259 (94.415, -26.1611) -> (90.4151, -26.1615)
  spline S172 degree 3 poles (90.4151, -26.1615) (90.139, -26.1619) (89.9151, -26.3858) (89.9151, -26.6615) knots 0 0 0 0 1 1 1 1
  line L260 (89.9151, -26.6615) -> (89.9151, -39.6623)
  spline S173 degree 3 poles (89.9151, -39.6623) (89.9151, -39.938) (90.139, -40.1619) (90.4151, -40.1624) knots 0 0 0 0 1 1 1 1
  line L261 (90.4151, -40.1624) -> (94.415, -40.1629)
  line L262 (94.415, -40.1629) -> (94.4151, -40.6625)
  spline S174 degree 3 poles (94.4151, -40.6625) (94.4151, -40.9381) (94.639, -41.1619) (94.9151, -41.1625) knots 0 0 0 0 1 1 1 1
  line L263 (94.9151, -41.1625) -> (98.9151, -41.1625)
  spline S175 degree 3 poles (98.9151, -41.1625) (99.1912, -41.162) (99.4151, -40.9381) (99.4151, -40.6624) knots 0 0 0 0 1 1 1 1
  line L264 (61.3151, -40.6624) -> (61.3152, -40.1629)
  line L265 (61.3152, -40.1629) -> (65.3151, -40.1623)
  spline S176 degree 3 poles (65.3151, -40.1623) (65.5913, -40.1618) (65.8151, -39.938) (65.8152, -39.6623) knots 0 0 0 0 1 1 1 1
  line L266 (65.8152, -39.6623) -> (65.8152, -26.6615)
  spline S177 degree 3 poles (65.8152, -26.6615) (65.8151, -26.3858) (65.5913, -26.1619) (65.3151, -26.1615) knots 0 0 0 0 1 1 1 1
  line L267 (65.3151, -26.1615) -> (61.3152, -26.1611)
  line L268 (61.3152, -26.1611) -> (61.3151, -25.6615)
  spline S178 degree 3 poles (61.3151, -25.6615) (61.3151, -25.3858) (61.0912, -25.1619) (60.8151, -25.1614) knots 0 0 0 0 1 1 1 1
  line L269 (60.8151, -25.1614) -> (56.8151, -25.1614)
  spline S179 degree 3 poles (56.8151, -25.1614) (56.539, -25.1619) (56.3151, -25.3858) (56.3151, -25.6615) knots 0 0 0 0 1 1 1 1
  line L270 (56.3151, -25.6615) -> (56.3151, -26.1611)
  line L271 (56.3151, -26.1611) -> (52.3151, -26.1615)
  spline S180 degree 3 poles (52.3151, -26.1615) (52.039, -26.1619) (51.8151, -26.3858) (51.8151, -26.6615) knots 0 0 0 0 1 1 1 1
  line L272 (51.8151, -26.6615) -> (51.8151, -39.6623)
  spline S181 degree 3 poles (51.8151, -39.6623) (51.8151, -39.938) (52.039, -40.1619) (52.3151, -40.1624) knots 0 0 0 0 1 1 1 1
  line L273 (52.3151, -40.1624) -> (56.3151, -40.1629)
  line L274 (56.3151, -40.1629) -> (56.3151, -40.6625)
  spline S182 degree 3 poles (56.3151, -40.6625) (56.3151, -40.9381) (56.539, -41.1619) (56.8151, -41.1625) knots 0 0 0 0 1 1 1 1
  line L275 (56.8151, -41.1625) -> (60.8151, -41.1625)
  spline S183 degree 3 poles (60.8151, -41.1625) (61.0912, -41.162) (61.3151, -40.9381) (61.3151, -40.6624) knots 0 0 0 0 1 1 1 1
  line L276 (80.3651, -38.2812) -> (80.3652, -37.7816)
  line L277 (80.3652, -37.7816) -> (84.3651, -37.7811)
  spline S184 degree 3 poles (84.3651, -37.7811) (84.6413, -37.7805) (84.8651, -37.5567) (84.8652, -37.281) knots 0 0 0 0 1 1 1 1
  line L278 (84.8652, -37.281) -> (84.8652, -24.2803)
  spline S185 degree 3 poles (84.8652, -24.2803) (84.8651, -24.0045) (84.6413, -23.7806) (84.3651, -23.7803) knots 0 0 0 0 1 1 1 1
  line L279 (84.3651, -23.7803) -> (80.3652, -23.7799)
  line L280 (80.3652, -23.7799) -> (80.3651, -23.2802)
  spline S186 degree 3 poles (80.3651, -23.2802) (80.3651, -23.0045) (80.1412, -22.7806) (79.8651, -22.7802) knots 0 0 0 0 1 1 1 1
  line L281 (79.8651, -22.7802) -> (75.8651, -22.7802)
  spline S187 degree 3 poles (75.8651, -22.7802) (75.589, -22.7806) (75.3651, -23.0045) (75.3651, -23.2802) knots 0 0 0 0 1 1 1 1
  line L282 (75.3651, -23.2802) -> (75.365, -23.7799)
  line L283 (75.365, -23.7799) -> (71.3651, -23.7803)
  spline S188 degree 3 poles (71.3651, -23.7803) (71.089, -23.7806) (70.8651, -24.0045) (70.8651, -24.2803) knots 0 0 0 0 1 1 1 1
  line L284 (70.8651, -24.2803) -> (70.8651, -37.2811)
  spline S189 degree 3 poles (70.8651, -37.2811) (70.8651, -37.5568) (71.089, -37.7806) (71.3651, -37.7811) knots 0 0 0 0 1 1 1 1
  line L285 (71.3651, -37.7811) -> (75.365, -37.7817)
  line L286 (75.365, -37.7817) -> (75.3651, -38.2812)
  spline S190 degree 3 poles (75.3651, -38.2812) (75.3651, -38.5568) (75.589, -38.7807) (75.8651, -38.7812) knots 0 0 0 0 1 1 1 1
  line L287 (75.8651, -38.7812) -> (79.8651, -38.7812)
  spline S191 degree 3 poles (79.8651, -38.7812) (80.1412, -38.7807) (80.3651, -38.5568) (80.3651, -38.2812) knots 0 0 0 0 1 1 1 1
  line L288 (42.2651, -26.3749) -> (42.2652, -25.8754)
  line L289 (42.2652, -25.8754) -> (46.2651, -25.8749)
  spline S192 degree 3 poles (46.2651, -25.8749) (46.5413, -25.8744) (46.7651, -25.6505) (46.7652, -25.3748) knots 0 0 0 0 1 1 1 1
  line L290 (46.7652, -25.3748) -> (46.7652, -12.374)
  spline S193 degree 3 poles (46.7652, -12.374) (46.7651, -12.0983) (46.5413, -11.8744) (46.2651, -11.874) knots 0 0 0 0 1 1 1 1
  line L291 (46.2651, -11.874) -> (42.2652, -11.8736)
  line L292 (42.2652, -11.8736) -> (42.2651, -11.374)
  spline S194 degree 3 poles (42.2651, -11.374) (42.2651, -11.0983) (42.0412, -10.8744) (41.7651, -10.8739) knots 0 0 0 0 1 1 1 1
  line L293 (41.7651, -10.8739) -> (37.7651, -10.8739)
  spline S195 degree 3 poles (37.7651, -10.8739) (37.489, -10.8744) (37.2651, -11.0983) (37.2651, -11.374) knots 0 0 0 0 1 1 1 1
  line L294 (37.2651, -11.374) -> (37.2651, -11.8736)
  line L295 (37.2651, -11.8736) -> (33.2651, -11.874)
  spline S196 degree 3 poles (33.2651, -11.874) (32.989, -11.8744) (32.7651, -12.0983) (32.7651, -12.374) knots 0 0 0 0 1 1 1 1
  line L296 (32.7651, -12.374) -> (32.7651, -25.3748)
  spline S197 degree 3 poles (32.7651, -25.3748) (32.7651, -25.6505) (32.989, -25.8744) (33.2651, -25.8749) knots 0 0 0 0 1 1 1 1
  line L297 (33.2651, -25.8749) -> (37.2651, -25.8754)
  line L298 (37.2651, -25.8754) -> (37.2651, -26.3749)
  spline S198 degree 3 poles (37.2651, -26.3749) (37.2651, -26.6505) (37.489, -26.8744) (37.7651, -26.8749) knots 0 0 0 0 1 1 1 1
  line L299 (37.7651, -26.8749) -> (41.7651, -26.8749)
  spline S199 degree 3 poles (41.7651, -26.8749) (42.0412, -26.8744) (42.2651, -26.6505) (42.2651, -26.3749) knots 0 0 0 0 1 1 1 1
  spline S200 degree 3 poles (17.9526, -26.8749) (18.2288, -26.8744) (18.4526, -26.6505) (18.4526, -26.3749) knots 0 0 0 0 1 1 1 1
  line L300 (18.4526, -26.3749) -> (18.4526, -25.8754)
  line L301 (18.4526, -25.8754) -> (22.4526, -25.8749)
  spline S201 degree 3 poles (22.4526, -25.8749) (22.7287, -25.8744) (22.9526, -25.6505) (22.9526, -25.3748) knots 0 0 0 0 1 1 1 1
  line L302 (22.9526, -25.3748) -> (22.9526, -12.374)
  spline S202 degree 3 poles (22.9526, -12.374) (22.9526, -12.0983) (22.7287, -11.8744) (22.4526, -11.874) knots 0 0 0 0 1 1 1 1
  line L303 (22.4526, -11.874) -> (18.4526, -11.8736)
  line L304 (18.4526, -11.8736) -> (18.4526, -11.374)
  spline S203 degree 3 poles (18.4526, -11.374) (18.4526, -11.0983) (18.2287, -10.8744) (17.9526, -10.8739) knots 0 0 0 0 1 1 1 1
  line L305 (17.9526, -10.8739) -> (13.9526, -10.8739)
  spline S204 degree 3 poles (13.9526, -10.8739) (13.6765, -10.8744) (13.4526, -11.0983) (13.4526, -11.374) knots 0 0 0 0 1 1 1 1
  line L306 (13.4526, -11.374) -> (13.4526, -11.8736)
  line L307 (13.4526, -11.8736) -> (9.4526, -11.874)
  spline S205 degree 3 poles (9.4526, -11.874) (9.1765, -11.8744) (8.9526, -12.0983) (8.9526, -12.374) knots 0 0 0 0 1 1 1 1
  line L308 (8.9526, -12.374) -> (8.9526, -25.3748)
  spline S206 degree 3 poles (8.9526, -25.3748) (8.9526, -25.6505) (9.1765, -25.8744) (9.4526, -25.8749) knots 0 0 0 0 1 1 1 1
  line L309 (9.4526, -25.8749) -> (13.4526, -25.8754)
  line L310 (13.4526, -25.8754) -> (13.4526, -26.3749)
  spline S207 degree 3 poles (13.4526, -26.3749) (13.4526, -26.6505) (13.6765, -26.8744) (13.9526, -26.8749) knots 0 0 0 0 1 1 1 1
  line L311 (13.9526, -26.8749) -> (17.9526, -26.8749)
  line L312 (118.4651, -23.9937) -> (118.4652, -23.4941)
  line L313 (118.4652, -23.4941) -> (122.4651, -23.4936)
  spline S208 degree 3 poles (122.4651, -23.4936) (122.7413, -23.4932) (122.9651, -23.2693) (122.9652, -22.9936) knots 0 0 0 0 1 1 1 1
  line L314 (122.9652, -22.9936) -> (122.9652, -9.9928)
  spline S209 degree 3 poles (122.9652, -9.9928) (122.9651, -9.717) (122.7413, -9.4932) (122.4651, -9.4928) knots 0 0 0 0 1 1 1 1
  line L315 (122.4651, -9.4928) -> (118.4652, -9.4924)
  line L316 (118.4652, -9.4924) -> (118.4651, -8.9927)
  spline S210 degree 3 poles (118.4651, -8.9927) (118.4651, -8.717) (118.2412, -8.4931) (117.9651, -8.4927) knots 0 0 0 0 1 1 1 1
  line L317 (117.9651, -8.4927) -> (113.9651, -8.4927)
  spline S211 degree 3 poles (113.9651, -8.4927) (113.689, -8.4931) (113.4651, -8.717) (113.4651, -8.9927) knots 0 0 0 0 1 1 1 1
  line L318 (113.4651, -8.9927) -> (113.4651, -9.4924)
  line L319 (113.4651, -9.4924) -> (109.4651, -9.4928)
  spline S212 degree 3 poles (109.4651, -9.4928) (109.189, -9.4931) (108.9651, -9.717) (108.9651, -9.9928) knots 0 0 0 0 1 1 1 1
  line L320 (108.9651, -9.9928) -> (108.9651, -22.9936)
  spline S213 degree 3 poles (108.9651, -22.9936) (108.9651, -23.2693) (109.189, -23.4931) (109.4651, -23.4936) knots 0 0 0 0 1 1 1 1
  line L321 (109.4651, -23.4936) -> (113.4651, -23.4941)
  line L322 (113.4651, -23.4941) -> (113.4651, -23.9937)
  spline S214 degree 3 poles (113.4651, -23.9937) (113.4651, -24.2693) (113.689, -24.4931) (113.9651, -24.4937) knots 0 0 0 0 1 1 1 1
  line L323 (113.9651, -24.4937) -> (117.9651, -24.4937)
  spline S215 degree 3 poles (117.9651, -24.4937) (118.2412, -24.4931) (118.4651, -24.2693) (118.4651, -23.9937) knots 0 0 0 0 1 1 1 1
  line L324 (99.4151, -21.6124) -> (99.4152, -21.1129)
  line L325 (99.4152, -21.1129) -> (103.4151, -21.1124)
  spline S216 degree 3 poles (103.4151, -21.1124) (103.6913, -21.1119) (103.9151, -20.888) (103.9152, -20.6123) knots 0 0 0 0 1 1 1 1
  line L326 (103.9152, -20.6123) -> (103.9152, -7.6115)
  spline S217 degree 3 poles (103.9152, -7.6115) (103.9151, -7.3358) (103.6913, -7.1119) (103.4151, -7.1115) knots 0 0 0 0 1 1 1 1
  line L327 (103.4151, -7.1115) -> (99.4152, -7.1111)
  line L328 (99.4152, -7.1111) -> (99.4151, -6.6115)
  spline S218 degree 3 poles (99.4151, -6.6115) (99.4151, -6.3358) (99.1912, -6.1119) (98.9151, -6.1114) knots 0 0 0 0 1 1 1 1
  line L329 (98.9151, -6.1114) -> (94.9151, -6.1114)
  spline S219 degree 3 poles (94.9151, -6.1114) (94.639, -6.1119) (94.4151, -6.3358) (94.4151, -6.6115) knots 0 0 0 0 1 1 1 1
  line L330 (94.4151, -6.6115) -> (94.415, -7.1111)
  line L331 (94.415, -7.1111) -> (90.4151, -7.1115)
  spline S220 degree 3 poles (90.4151, -7.1115) (90.139, -7.1119) (89.9151, -7.3358) (89.9151, -7.6115) knots 0 0 0 0 1 1 1 1
  line L332 (89.9151, -7.6115) -> (89.9151, -20.6123)
  spline S221 degree 3 poles (89.9151, -20.6123) (89.9151, -20.888) (90.139, -21.1119) (90.4151, -21.1124) knots 0 0 0 0 1 1 1 1
  line L333 (90.4151, -21.1124) -> (94.415, -21.1129)
  line L334 (94.415, -21.1129) -> (94.4151, -21.6124)
  spline S222 degree 3 poles (94.4151, -21.6124) (94.4151, -21.888) (94.639, -22.1119) (94.9151, -22.1124) knots 0 0 0 0 1 1 1 1
  line L335 (94.9151, -22.1124) -> (98.9151, -22.1124)
  spline S223 degree 3 poles (98.9151, -22.1124) (99.1912, -22.1119) (99.4151, -21.888) (99.4151, -21.6124) knots 0 0 0 0 1 1 1 1
  line L336 (61.3151, -21.6124) -> (61.3152, -21.1129)
  line L337 (61.3152, -21.1129) -> (65.3151, -21.1124)
  spline S224 degree 3 poles (65.3151, -21.1124) (65.5913, -21.1119) (65.8151, -20.888) (65.8152, -20.6123) knots 0 0 0 0 1 1 1 1
  line L338 (65.8152, -20.6123) -> (65.8152, -7.6115)
  spline S225 degree 3 poles (65.8152, -7.6115) (65.8151, -7.3358) (65.5913, -7.1119) (65.3151, -7.1115) knots 0 0 0 0 1 1 1 1
  line L339 (65.3151, -7.1115) -> (61.3152, -7.1111)
  line L340 (61.3152, -7.1111) -> (61.3151, -6.6115)
  spline S226 degree 3 poles (61.3151, -6.6115) (61.3151, -6.3358) (61.0912, -6.1119) (60.8151, -6.1114) knots 0 0 0 0 1 1 1 1
  line L341 (60.8151, -6.1114) -> (56.8151, -6.1114)
  spline S227 degree 3 poles (56.8151, -6.1114) (56.539, -6.1119) (56.3151, -6.3358) (56.3151, -6.6115) knots 0 0 0 0 1 1 1 1
  line L342 (56.3151, -6.6115) -> (56.3151, -7.1111)
  line L343 (56.3151, -7.1111) -> (52.3151, -7.1115)
  spline S228 degree 3 poles (52.3151, -7.1115) (52.039, -7.1119) (51.8151, -7.3358) (51.8151, -7.6115) knots 0 0 0 0 1 1 1 1
  line L344 (51.8151, -7.6115) -> (51.8151, -20.6123)
  spline S229 degree 3 poles (51.8151, -20.6123) (51.8151, -20.888) (52.039, -21.1119) (52.3151, -21.1124) knots 0 0 0 0 1 1 1 1
  line L345 (52.3151, -21.1124) -> (56.3151, -21.1129)
  line L346 (56.3151, -21.1129) -> (56.3151, -21.6124)
  spline S230 degree 3 poles (56.3151, -21.6124) (56.3151, -21.888) (56.539, -22.1119) (56.8151, -22.1124) knots 0 0 0 0 1 1 1 1
  line L347 (56.8151, -22.1124) -> (60.8151, -22.1124)
  spline S231 degree 3 poles (60.8151, -22.1124) (61.0912, -22.1119) (61.3151, -21.888) (61.3151, -21.6124) knots 0 0 0 0 1 1 1 1
  line L348 (80.3651, -19.2312) -> (80.3652, -18.7316)
  line L349 (80.3652, -18.7316) -> (84.3651, -18.7311)
  spline S232 degree 3 poles (84.3651, -18.7311) (84.6413, -18.7307) (84.8651, -18.5068) (84.8652, -18.2311) knots 0 0 0 0 1 1 1 1
  line L350 (84.8652, -18.2311) -> (84.8652, -5.2303)
  spline S233 degree 3 poles (84.8652, -5.2303) (84.8651, -4.9545) (84.6413, -4.7307) (84.3651, -4.7303) knots 0 0 0 0 1 1 1 1